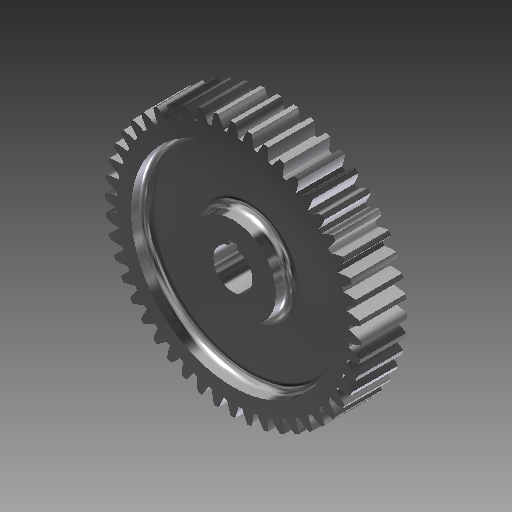
# Autodesk Inventor part: Spur Gear1
Saved by Autodesk Inventor 2020 (Build 240168000, 168)
## iProperties
CustomPartVersion: 1
Created: 2016-04-28
Part Number: Spur Gear1
Material: Steel, Cast
Document SubType Name: Modeling
Designer: Jorge
Categories: <?xml version="1.0" encoding="UTF-16"?> <MemberInstance><Categories><FamilyTemplate><FamilyTemplateParameter ValueType="xs:double" Id="1" ObjectReferenceKey="da_z" ObjectType="kUserParameterObject"/><FamilyTemplateParameter ValueType="xs:double" Id="2" ObjectReferenceKey="da_b" ObjectType="kUserParameterObject"/><FamilyTemplateParameter ValueType="xs:double" Id="3" ObjectReferenceKey="da_beta" ObjectType="kUserParameterObject"/><FamilyTemplateParameter ValueType="xs:double" Id="4" ObjectReferenceKey="da_da" ObjectType="kUserParameterObject"/><FamilyTemplateParameter ValueType="xs:double" Id="5" ObjectReferenceKey="da_aw" ObjectType="kUserParameterObject"/><FamilyTemplateParameter ValueType="xs:string" Id="6" ObjectReferenceKey="EAIAABAAAAC/AAAAAAAAAIAAAAAAAAAA" ObjectType="83910656" SubObjectId="SurfaceGeometry"/></FamilyTemplate><ParamToTemplateMap><ParamToTemplate CategoryParameter="//CategoryParameter[@InternalName='046C89C9-8512-4d59-83FE-43B91F4F132A']" TemplateParameter="1"/><ParamToTemplate CategoryParameter="//CategoryParameter[@InternalName='2552DF32-E462-4b46-AEBF-C6C7768E72AC']" TemplateParameter="2"/><ParamToTemplate CategoryParameter="//CategoryParameter[@InternalName='C9EE641D-15FC-4fae-A226-E94C4372FDD7']" TemplateParameter="3"/><ParamToTemplate><ParamToTemplate CategoryParameter="//CategoryParameter[@InternalName='00B6519A-459B-49c7-AD84-2E56D39A5744']" ConstantValue="-0.500000"/></ParamToTemplate><ParamToTemplate><ParamToTemplate CategoryParameter="//CategoryParameter[@InternalName='04B31F0E-C7A6-4894-AA32-9629BEFACF47']" ConstantValue="1.000000"/></ParamToTemplate><ParamToTemplate><ParamToTemplate CategoryParameter="//CategoryParameter[@InternalName='43CBEC2E-7847-49e7-A936-2F7889FCB2D9']" ConstantValue="0.250000"/></ParamToTemplate><ParamToTemplate><ParamToTemplate CategoryParameter="//CategoryParameter[@InternalName='B1EFC894-105D-4ebd-86BF-FA20ED196853']" ConstantValue="0.333500"/></ParamToTemplate><ParamToTemplate><ParamToTemplate CategoryParameter="//CategoryParameter[@InternalName='51175063-3D10-4879-93E8-6246FE8B403D']" ConstantValue="2061532430.657340"/></ParamToTemplate><ParamToTemplate><ParamToTemplate CategoryParameter="//CategoryParameter[@InternalName='A3A52E27-4454-46a9-B0BD-C932399B70AF']" ConstantValue="0.300000"/></ParamToTemplate><ParamToTemplate><ParamToTemplate CategoryParameter="//CategoryParameter[@InternalName='91B76062-C214-41d9-B1B9-14D2AB99603D']" ConstantValue="0.211667"/></ParamToTemplate><ParamToTemplate><ParamToTemplate CategoryParameter="//CategoryParameter[@InternalName='374E806E-8B8A-4dda-A9AA-1039D6500AD2']" ConstantValue="4.724409"/></ParamToTemplate><ParamToTemplate><ParamToTemplate CategoryParameter="//CategoryParameter[@InternalName='2D373A89-B862-43d6-8D0B-0CBF12AB9F6C']" ConstantValue="0.253073"/></ParamToTemplate><ParamToTemplate CategoryParameter="//CategoryParameter[@InternalName='37777632-D6A2-4fac-9D53-DB8ACD95C989']" TemplateParameter="4"/><ParamToTemplate CategoryParameter="//CategoryParameter[@InternalName='FD1017F1-B727-4f7e-9707-0F86F1FF9423']" TemplateParameter="5"/><ParamToTemplate><ParamToTemplate CategoryParameter="//CategoryParameter[@InternalName='9E1B4470-B2D3-4ff1-B813-535BB4CDF51A']" ConstantValue="3523220.976809"/></ParamToTemplate><ParamToTemplate><ParamToTemplate CategoryParameter="//CategoryParameter[@InternalName='F8452263-BFF6-458c-9FB1-07C4B99E95CD']" ConstantValue="11397033.805607"/></ParamToTemplate><ParamToTemplate><ParamToTemplate CategoryParameter="//CategoryParameter[@InternalName='3E3BB259-FD49-497f-8171-6EBC954A3479']" ConstantValue="2.000000"/></ParamToTemplate><ParamToTemplate CategoryParameter="//CategoryParameter[@InternalName='27C3BAF2-7550-4e4b-AE2C-0DB134B7D9B7']" TemplateParameter="6"/></ParamToTemplateMap><Category DisplayName="Gear" InternalName="DC85795E-93AB-48d5-8EEE-5A27447B64BD" Mnemonic="Gear"><CategoryParameter DisplayName="z" InternalName="046C89C9-8512-4d59-83FE-43B91F4F132A" Mnemonic="z"/><CategoryParameter DisplayName="b" InternalName="2552DF32-E462-4b46-AEBF-C6C7768E72AC" Mnemonic="b"/><CategoryParameter DisplayName="||b|" InternalName="C9EE641D-15FC-4fae-A226-E94C4372FDD7" Mnemonic="beta"/><CategoryParameter DisplayName="x" InternalName="00B6519A-459B-49c7-AD84-2E56D39A5744" Mnemonic="x"/><CategoryParameter DisplayName="a*" InternalName="04B31F0E-C7A6-4894-AA32-9629BEFACF47" Mnemonic="a"/><CategoryParameter DisplayName="c*" InternalName="43CBEC2E-7847-49e7-A936-2F7889FCB2D9" Mnemonic="c"/><CategoryParameter DisplayName="r|.f|*" InternalName="B1EFC894-105D-4ebd-86BF-FA20ED196853" Mnemonic="rf"/><CategoryParameter DisplayName="E" InternalName="51175063-3D10-4879-93E8-6246FE8B403D" Mnemonic="E"/><CategoryParameter DisplayName="||m|" InternalName="A3A52E27-4454-46a9-B0BD-C932399B70AF" Mnemonic="mi"/><Category DisplayName="SpurGear" InternalName="26C5A22E-A91E-4dfd-A3B3-23CCAFAE1764" Mnemonic="SpurGear"><CategoryParameter DisplayName="m" InternalName="91B76062-C214-41d9-B1B9-14D2AB99603D" Mnemonic="m"/><CategoryParameter DisplayName="P" InternalName="374E806E-8B8A-4dda-A9AA-1039D6500AD2" Mnemonic="PP"/><CategoryParameter DisplayName="||a|" InternalName="2D373A89-B862-43d6-8D0B-0CBF12AB9F6C" Mnemonic="alpha"/><CategoryParameter DisplayName="d|.a|" InternalName="37777632-D6A2-4fac-9D53-DB8ACD95C989" Mnemonic="da"/><CategoryParameter DisplayName="a|.w|" InternalName="FD1017F1-B727-4f7e-9707-0F86F1FF9423" Mnemonic="aw"/><CategoryParameter DisplayName="||s||.Flim|" InternalName="9E1B4470-B2D3-4ff1-B813-535BB4CDF51A" Mnemonic="sFlim"/><CategoryParameter DisplayName="||s||.Hlim|" InternalName="F8452263-BFF6-458c-9FB1-07C4B99E95CD" Mnemonic="sHlim"/><CategoryParameter DisplayName="type" InternalName="3E3BB259-FD49-497f-8171-6EBC954A3479" Mnemonic="type"/><CategoryParameter DisplayName="PitchDiameter" InternalName="27C3BAF2-7550-4e4b-AE2C-0DB134B7D9B7" Mnemonic="IDS_PITCHDIAM"/></Category></Category></Categories></MemberInstance>
Density: 7.85 g/cm^3
Appearance: Semi-Polished
Mass: 685.005 g
Surface Area: 317.398 cm^2
Volume: 87.2617 cm^3
Author: Jorge
Autodesk Inventor part; units mm, degrees
sketch "Sketch1" plane through (0, 0, 0) normal (0, 0, 1) x (1, 0, 0)
  circle A0 centre (0, 0) radius 51.8534
  dimension "d0" = 103.7068
  constraints: 1 centre point
  measures "d0" diameter of A0
extrude "Extrusion1" add sketch "Sketch1" along normal blind 18.796
sketch "Sketch2" plane through (0, 0, 0) normal (0, 0, -1) x (-1, 0, 0)
  circle A0 centre (0, 0) radius 51.8534 projected
  circle A1 centre (0, 0) radius 50.9654
  dimension "d3" = 101.9308
  constraints: 1 centre point, 1 coincident
  measures "d3" diameter of A1
surface extrude "Pitch Diameter" sketch "Sketch2" against normal through all shown no curves A1
ref_plane "Work Plane1" through (0, 0, 0) normal (1, 0, 0) x (0, 1, 0)
ref_plane "Work Plane2" through (0, 0, 0) normal (0.9978589, 0.0654031, 0) x (0, 0, 1)
ref_plane "Work Plane3" through (0, 0, 9.398) normal (0, 0, -1) x (-1, 0, 0)
spur gear teeth "Spur Gear" teeth 48 pitch diameter 101.6 tip diameter 103.7068 root diameter 94.1917 face width 18.796 start plane through (0, 0, 0) normal (0, 0, -1) x (-1, 0, 0)
ref_plane "Work Plane4" through (0, 0, 9.398) normal (0, 0, 1) x (1, 0, 0)
sketch "Sketch3" plane through (0, 0, 0) normal (1, 0, 0) x (0, 1, 0)
  line L0 (41.275, 18.796) -> (17.4625, 18.796)
  line L1 (17.4625, 18.796) -> (17.4625, 15.621)
  line L2 (20.6375, 12.446) -> (38.1, 12.446)
  line L3 (41.275, 15.621) -> (41.275, 18.796)
  line L4 (0, -9.2156) -> (0, 55.2938) projected
  line L5 (12.5993, 18.796) -> (9.9425, 18.796) projected
  arc A0 (38.1, 12.446) -> (41.275, 15.621) centre (38.1, 15.621) ccw
  arc A1 (17.4625, 15.621) -> (20.6375, 12.446) centre (20.6375, 15.621) ccw
  line L6 (-72.5948, 9.398) -> (72.5948, 9.398) construction
  line L7 (41.275, 0) -> (17.4625, 0)
  line L8 (17.4625, 0) -> (17.4625, 3.175)
  line L9 (20.6375, 6.35) -> (38.1, 6.35)
  line L10 (41.275, 3.175) -> (41.275, 0)
  arc A2 (41.275, 3.175) -> (38.1, 6.35) centre (38.1, 3.175) ccw
  arc A3 (20.6375, 6.35) -> (17.4625, 3.175) centre (20.6375, 3.175) ccw
  point P0 (0, 0)
  dimension "d20" = 82.55
  dimension "d21" = 34.925
  dimension "d22" = 0
  dimension "d23" = 6.35
  dimension "d24" = 3.175
  constraints: 16 end point, 8 point on circle, 8 symmetric about line, 4 centre point, 4 tangent, 2 parallel, 1 equal radius, 1 horizontal, 1 perpendicular, 2 other
  measures "d20" diameter of L3 L4
  measures "d21" diameter of L1 L4
  measures "d22" distance between parallel lines of L5 L0
  measures "d23" distance between parallel lines of L2 L0
  measures "d24" radius of A0
revolve "Revolution1" cut sketch "Sketch3" angle 360 about axis through (0, 0, 0) along (0, 0, 1)
hole "Hole1" at (0, 0, 18.796) direction (0, 0, -1) diameter 15.8623 end through all
sketch "Sketch4" plane through (0, 0, 18.796) normal (0, 0, 1) x (1, 0, 0)
  line L0 (-1.5875, 6.3437) -> (1.5875, 6.3437)
  line L1 (1.5875, 6.3437) -> (1.5875, 9.5187)
  line L2 (1.5875, 9.5187) -> (-1.5875, 9.5187)
  line L3 (-1.5875, 9.5187) -> (-1.5875, 6.3437)
  circle A0 centre (0, 0) radius 7.9312 construction
  line L4 (0, 72.5948) -> (0, -72.5948) construction
  line L5 (-4.4972, 7.9312) -> (3.3185, 7.9312) construction
  dimension "d35" = 3.175
  dimension "d36" = 1.5875
  dimension "d37" = 1.5875
  dimension "d38" = 3.175
  constraints: 10 end point, 2 horizontal, 2 parallel, 1 perpendicular, 1 tangent
  measures "d35" distance between parallel lines of L1 L3
  measures "d36" distance between parallel lines of L4 L1
  measures "d37" distance between parallel lines of L2 L5
  measures "d38" distance between parallel lines of L2 L0
extrude "Extrusion2" cut sketch "Sketch4" against normal through all
equation "\"d0\" = da_da"
equation "\"d1\" = da_b"
equation "\"d3\" = da_dw"
equation "\"d36\" = 0.5 * d35"
equation "\"d38\" = 2 * d37"
equation "\"d15\" = da_aw"
equation "\"d19\" = da_aw"
equation "\"da_da\" = 103.706793"
equation "\"da_b\" = 18.796"
equation "\"da_dw\" = 101.930768"
equation "\"da_aw\" = 63.70673"
body "Solid1"
body "Srf1"
